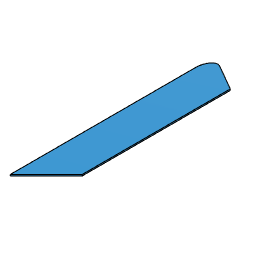
Nupud-T v2 (Autodesk Fusion 360 design; units mm, degrees)
Autodesk Fusion 360 part; units mm, degrees
sketch "Sketch1" plane through (0, 0, 0) normal (0, 0, 1) x (1, 0, 0)
  line L0 (50, -108) -> (50, -39.3754)
  line L1 (50, -39.3754) -> (38.2856, -32.6121)
  spline S0 degree 3 poles (38.2856, -32.6121) (37.4771, -32.1422) (36.6924, -32.1202) (35.8815, -32.5337) (35.0622, -32.9516) (34.2278, -33.9044) (33.6842, -35.2367) (33.2499, -36.3014) (33.0037, -37.5868) (33, -38.8754) knots -0.361367 -0.361367 -0.361367 -0.361367 0.324344 0.324344 0.324344 1.017159 1.017159 1.017159 1.570796 1.570796 1.570796 1.570796
  line L2 (33, -38.8754) -> (33, -125)
  line L3 (33, -125) -> (50, -108)
  line L4 (49.8, -107.9172) -> (49.8, -39.4909)
  line L5 (49.8, -39.4909) -> (38.1854, -32.7852)
  spline S1 degree 3 poles (38.1854, -32.7852) (38.1853, -32.7851) (38.1852, -32.7851) (38.1851, -32.785) (37.4228, -32.342) (36.7342, -32.3234) (35.9723, -32.7119) (35.2137, -33.0988) (34.3985, -34.0153) (33.8694, -35.3123) (33.4463, -36.3493) (33.2036, -37.6124) (33.2, -38.876) knots -0.361437 -0.361437 -0.361437 -0.361437 -0.361367 -0.361367 -0.361367 0.324344 0.324344 0.324344 1.017159 1.017159 1.017159 1.570796 1.570796 1.570796 1.570796
  line L6 (33.2, -38.876) -> (33.2, -124.5172)
  line L7 (33.2, -124.5172) -> (49.8, -107.9172)
  dimension "d1" = 45
  dimension "d2" = 17
  dimension "d3" = 33
  dimension "d4" = 125
  dimension "d5" = 120
  dimension "d6" = 0.5
  dimension "d7" = -0.2
  constraint vertical L2
  constraint vertical L0
  measures "d1" angle of L2 L3
  measures "d2" distance of L0 L2
  measures "d3" distance of origin L2
  measures "d4" vertical distance of origin L2.end
  measures "d5" angle of L0 L1
  measures "d6" distance of L0.end S0.end
extrude "Extrude1" add sketch "Sketch1" along normal blind 0.6 contours L4 L5 S1 L6 L7
